Autodesk Fusion 360 part; units mm, degrees
(part 4 of 12)
  arc A1641 (188.5059, 15.9968) -> (187.8959, 15.9968) centre (188.2009, 15.9968) ccw
  arc A1642 (194.7044, 9.8652) -> (195.3144, 9.8652) centre (195.0094, 9.8652) ccw
  arc A1643 (195.3144, 9.8652) -> (194.7044, 9.8652) centre (195.0094, 9.8652) ccw
  arc A1644 (37.157, 59.1472) -> (37.767, 59.1472) centre (37.462, 59.1472) ccw
  arc A1645 (37.767, 59.1472) -> (37.157, 59.1472) centre (37.462, 59.1472) ccw
  arc A1646 (172.2547, 3.3052) -> (171.6447, 3.3052) centre (171.9497, 3.3052) ccw
  arc A1647 (171.6447, 3.3052) -> (172.2547, 3.3052) centre (171.9497, 3.3052) ccw
  arc A1648 (19.3498, 20.1403) -> (19.9598, 20.1403) centre (19.6548, 20.1403) ccw
  arc A1649 (19.9598, 20.1403) -> (19.3498, 20.1403) centre (19.6548, 20.1403) ccw
  arc A1650 (196.076, 32.2079) -> (196.686, 32.2079) centre (196.381, 32.2079) ccw
  arc A1651 (196.686, 32.2079) -> (196.076, 32.2079) centre (196.381, 32.2079) ccw
  arc A1652 (65.3089, -31.7901) -> (65.9189, -31.7901) centre (65.6139, -31.7901) ccw
  arc A1653 (65.9189, -31.7901) -> (65.3089, -31.7901) centre (65.6139, -31.7901) ccw
  arc A1654 (100.1137, 28.1421) -> (99.5037, 28.1421) centre (99.8087, 28.1421) ccw
  arc A1655 (99.5037, 28.1421) -> (100.1137, 28.1421) centre (99.8087, 28.1421) ccw
  arc A1656 (38.7626, 74.6874) -> (39.3726, 74.6874) centre (39.0676, 74.6874) ccw
  arc A1657 (39.3726, 74.6874) -> (38.7626, 74.6874) centre (39.0676, 74.6874) ccw
  arc A1658 (68.1725, 81.757) -> (68.7825, 81.757) centre (68.4775, 81.757) ccw
  arc A1659 (68.7825, 81.757) -> (68.1725, 81.757) centre (68.4775, 81.757) ccw
  arc A1660 (98.8111, 74.853) -> (99.4211, 74.853) centre (99.1161, 74.853) ccw
  arc A1661 (99.4211, 74.853) -> (98.8111, 74.853) centre (99.1161, 74.853) ccw
  arc A1662 (129.2833, 80.5774) -> (129.8933, 80.5774) centre (129.5883, 80.5774) ccw
  arc A1663 (129.8933, 80.5774) -> (129.2833, 80.5774) centre (129.5883, 80.5774) ccw
  arc A1664 (158.9828, 74.2089) -> (159.5928, 74.2089) centre (159.2878, 74.2089) ccw
  arc A1665 (159.5928, 74.2089) -> (158.9828, 74.2089) centre (159.2878, 74.2089) ccw
  arc A1666 (194.1649, 74.2089) -> (194.7749, 74.2089) centre (194.4699, 74.2089) ccw
  arc A1667 (194.7749, 74.2089) -> (194.1649, 74.2089) centre (194.4699, 74.2089) ccw
  arc A1668 (191.6955, 42.1421) -> (192.3055, 42.1421) centre (192.0005, 42.1421) ccw
  arc A1669 (192.3055, 42.1421) -> (191.6955, 42.1421) centre (192.0005, 42.1421) ccw
  arc A1670 (214.7839, 42.1421) -> (215.3939, 42.1421) centre (215.0889, 42.1421) ccw
  arc A1671 (215.3939, 42.1421) -> (214.7839, 42.1421) centre (215.0889, 42.1421) ccw
  arc A1672 (74.5184, 16.8462) -> (73.9084, 16.8462) centre (74.2134, 16.8462) ccw
  arc A1673 (73.9084, 16.8462) -> (74.5184, 16.8462) centre (74.2134, 16.8462) ccw
  arc A1674 (109.4184, 19.9249) -> (110.0284, 19.9249) centre (109.7234, 19.9249) ccw
  arc A1675 (110.0284, 19.9249) -> (109.4184, 19.9249) centre (109.7234, 19.9249) ccw
  arc A1676 (180.1512, -15.9405) -> (180.7612, -15.9405) centre (180.4562, -15.9405) ccw
  arc A1677 (180.7612, -15.9405) -> (180.1512, -15.9405) centre (180.4562, -15.9405) ccw
  arc A1678 (206.6439, -9.7413) -> (207.2539, -9.7413) centre (206.9489, -9.7413) ccw
  arc A1679 (207.2539, -9.7413) -> (206.6439, -9.7413) centre (206.9489, -9.7413) ccw
  arc A1680 (100.8626, -25.7268) -> (101.4726, -25.7268) centre (101.1676, -25.7268) ccw
  arc A1681 (101.4726, -25.7268) -> (100.8626, -25.7268) centre (101.1676, -25.7268) ccw
  line L279 (39.8781, 79.4042) -> (43.6781, 79.4042)
  line L280 (43.6781, 79.4042) -> (43.6781, 75.6042)
  line L281 (43.6781, 75.6042) -> (39.8781, 75.6042)
  line L282 (39.8781, 75.6042) -> (39.8781, 79.4042)
  arc A1682 (39.6622, 82.1982) -> (43.65, 82.1982) centre (41.6561, 82.1982) ccw
  arc A1683 (43.65, 82.1982) -> (39.6622, 82.1982) centre (41.6561, 82.1982) ccw
  arc A1684 (47.587, 82.0712) -> (45.8852, 82.0712) centre (46.7361, 82.0712) ccw
  arc A1685 (45.8852, 82.0712) -> (47.587, 82.0712) centre (46.7361, 82.0712) ccw
  arc A1686 (37.427, 82.0712) -> (35.7252, 82.0712) centre (36.5761, 82.0712) ccw
  arc A1687 (35.7252, 82.0712) -> (37.427, 82.0712) centre (36.5761, 82.0712) ccw
  line L283 (69.8781, 79.4042) -> (73.6781, 79.4042)
  line L284 (69.8781, 75.6042) -> (69.8781, 79.4042)
  line L285 (73.6781, 75.6042) -> (69.8781, 75.6042)
  line L286 (73.6781, 79.4042) -> (73.6781, 75.6042)
  arc A1688 (69.6622, 82.1982) -> (73.65, 82.1982) centre (71.6561, 82.1982) ccw
  arc A1689 (73.65, 82.1982) -> (69.6622, 82.1982) centre (71.6561, 82.1982) ccw
  arc A1690 (75.8852, 82.0712) -> (77.587, 82.0712) centre (76.7361, 82.0712) ccw
  arc A1691 (77.587, 82.0712) -> (75.8852, 82.0712) centre (76.7361, 82.0712) ccw
  arc A1692 (65.7252, 82.0712) -> (67.427, 82.0712) centre (66.5761, 82.0712) ccw
  arc A1693 (67.427, 82.0712) -> (65.7252, 82.0712) centre (66.5761, 82.0712) ccw
  line L287 (99.8781, 79.4042) -> (103.6781, 79.4042)
  line L288 (103.6781, 79.4042) -> (103.6781, 75.6042)
  line L289 (103.6781, 75.6042) -> (99.8781, 75.6042)
  line L290 (99.8781, 75.6042) -> (99.8781, 79.4042)
  arc A1694 (99.6622, 82.1982) -> (103.65, 82.1982) centre (101.6561, 82.1982) ccw
  arc A1695 (103.65, 82.1982) -> (99.6622, 82.1982) centre (101.6561, 82.1982) ccw
  arc A1696 (105.8852, 82.0712) -> (107.587, 82.0712) centre (106.7361, 82.0712) ccw
  arc A1697 (107.587, 82.0712) -> (105.8852, 82.0712) centre (106.7361, 82.0712) ccw
  arc A1698 (95.7252, 82.0712) -> (97.427, 82.0712) centre (96.5761, 82.0712) ccw
  arc A1699 (97.427, 82.0712) -> (95.7252, 82.0712) centre (96.5761, 82.0712) ccw
  line L291 (133.6781, 79.4042) -> (133.6781, 75.6042)
  line L292 (133.6781, 75.6042) -> (129.8781, 75.6042)
  line L293 (129.8781, 75.6042) -> (129.8781, 79.4042)
  line L294 (129.8781, 79.4042) -> (133.6781, 79.4042)
  arc A1700 (129.6622, 82.1982) -> (133.65, 82.1982) centre (131.6561, 82.1982) ccw
  arc A1701 (133.65, 82.1982) -> (129.6622, 82.1982) centre (131.6561, 82.1982) ccw
  arc A1702 (135.8852, 82.0712) -> (137.587, 82.0712) centre (136.7361, 82.0712) ccw
  arc A1703 (137.587, 82.0712) -> (135.8852, 82.0712) centre (136.7361, 82.0712) ccw
  arc A1704 (125.7252, 82.0712) -> (127.427, 82.0712) centre (126.5761, 82.0712) ccw
  arc A1705 (127.427, 82.0712) -> (125.7252, 82.0712) centre (126.5761, 82.0712) ccw
  line L295 (159.8781, 79.4042) -> (163.6781, 79.4042)
  line L296 (163.6781, 79.4042) -> (163.6781, 75.6042)
  line L297 (163.6781, 75.6042) -> (159.8781, 75.6042)
  line L298 (159.8781, 75.6042) -> (159.8781, 79.4042)
  arc A1706 (159.6622, 82.1982) -> (163.65, 82.1982) centre (161.6561, 82.1982) ccw
  arc A1707 (163.65, 82.1982) -> (159.6622, 82.1982) centre (161.6561, 82.1982) ccw
  arc A1708 (165.8852, 82.0712) -> (167.587, 82.0712) centre (166.7361, 82.0712) ccw
  arc A1709 (167.587, 82.0712) -> (165.8852, 82.0712) centre (166.7361, 82.0712) ccw
  arc A1710 (157.427, 82.0712) -> (155.7252, 82.0712) centre (156.5761, 82.0712) ccw
  arc A1711 (155.7252, 82.0712) -> (157.427, 82.0712) centre (156.5761, 82.0712) ccw
  line L299 (193.6781, 79.4042) -> (193.6781, 75.6042)
  line L300 (193.6781, 75.6042) -> (189.8781, 75.6042)
  line L301 (189.8781, 75.6042) -> (189.8781, 79.4042)
  line L302 (189.8781, 79.4042) -> (193.6781, 79.4042)
  arc A1712 (189.6622, 82.1982) -> (193.65, 82.1982) centre (191.6561, 82.1982) ccw
  arc A1713 (193.65, 82.1982) -> (189.6622, 82.1982) centre (191.6561, 82.1982) ccw
  arc A1714 (195.8852, 82.0712) -> (197.587, 82.0712) centre (196.7361, 82.0712) ccw
  arc A1715 (197.587, 82.0712) -> (195.8852, 82.0712) centre (196.7361, 82.0712) ccw
  arc A1716 (187.427, 82.0712) -> (185.7252, 82.0712) centre (186.5761, 82.0712) ccw
  arc A1717 (185.7252, 82.0712) -> (187.427, 82.0712) centre (186.5761, 82.0712) ccw
  line L303 (223.6781, 75.6042) -> (219.8781, 75.6042)
  line L304 (219.8781, 75.6042) -> (219.8781, 79.4042)
  line L305 (223.6781, 79.4042) -> (223.6781, 75.6042)
  line L306 (219.8781, 79.4042) -> (223.6781, 79.4042)
  arc A1718 (219.6622, 82.1982) -> (223.65, 82.1982) centre (221.6561, 82.1982) ccw
  arc A1719 (223.65, 82.1982) -> (219.6622, 82.1982) centre (221.6561, 82.1982) ccw
  arc A1720 (225.8852, 82.0712) -> (227.587, 82.0712) centre (226.7361, 82.0712) ccw
  arc A1721 (227.587, 82.0712) -> (225.8852, 82.0712) centre (226.7361, 82.0712) ccw
  arc A1722 (215.7252, 82.0712) -> (217.427, 82.0712) centre (216.5761, 82.0712) ccw
  arc A1723 (217.427, 82.0712) -> (215.7252, 82.0712) centre (216.5761, 82.0712) ccw
  line L307 (39.8781, 49.4042) -> (43.6781, 49.4042)
  line L308 (43.6781, 49.4042) -> (43.6781, 45.6042)
  line L309 (43.6781, 45.6042) -> (39.8781, 45.6042)
  line L310 (39.8781, 45.6042) -> (39.8781, 49.4042)
  arc A1724 (43.65, 52.1982) -> (39.6622, 52.1982) centre (41.6561, 52.1982) ccw
  arc A1725 (39.6622, 52.1982) -> (43.65, 52.1982) centre (41.6561, 52.1982) ccw
  arc A1726 (45.8852, 52.0712) -> (47.587, 52.0712) centre (46.7361, 52.0712) ccw
  arc A1727 (47.587, 52.0712) -> (45.8852, 52.0712) centre (46.7361, 52.0712) ccw
  arc A1728 (35.7252, 52.0712) -> (37.427, 52.0712) centre (36.5761, 52.0712) ccw
  arc A1729 (37.427, 52.0712) -> (35.7252, 52.0712) centre (36.5761, 52.0712) ccw
  line L311 (69.8781, 49.4042) -> (73.6781, 49.4042)
  line L312 (73.6781, 49.4042) -> (73.6781, 45.6042)
  line L313 (69.8781, 45.6042) -> (69.8781, 49.4042)
  line L314 (73.6781, 45.6042) -> (69.8781, 45.6042)
  arc A1730 (69.6622, 52.1982) -> (73.65, 52.1982) centre (71.6561, 52.1982) ccw
  arc A1731 (73.65, 52.1982) -> (69.6622, 52.1982) centre (71.6561, 52.1982) ccw
  arc A1732 (75.8852, 52.0712) -> (77.587, 52.0712) centre (76.7361, 52.0712) ccw
  arc A1733 (77.587, 52.0712) -> (75.8852, 52.0712) centre (76.7361, 52.0712) ccw
  arc A1734 (65.7252, 52.0712) -> (67.427, 52.0712) centre (66.5761, 52.0712) ccw
  arc A1735 (67.427, 52.0712) -> (65.7252, 52.0712) centre (66.5761, 52.0712) ccw
  line L315 (99.8781, 45.6042) -> (99.8781, 49.4042)
  line L316 (99.8781, 49.4042) -> (103.6781, 49.4042)
  line L317 (103.6781, 49.4042) -> (103.6781, 45.6042)
  line L318 (103.6781, 45.6042) -> (99.8781, 45.6042)
  arc A1736 (99.6622, 52.1982) -> (103.65, 52.1982) centre (101.6561, 52.1982) ccw
  arc A1737 (103.65, 52.1982) -> (99.6622, 52.1982) centre (101.6561, 52.1982) ccw
  arc A1738 (105.8852, 52.0712) -> (107.587, 52.0712) centre (106.7361, 52.0712) ccw
  arc A1739 (107.587, 52.0712) -> (105.8852, 52.0712) centre (106.7361, 52.0712) ccw
  arc A1740 (95.7252, 52.0712) -> (97.427, 52.0712) centre (96.5761, 52.0712) ccw
  arc A1741 (97.427, 52.0712) -> (95.7252, 52.0712) centre (96.5761, 52.0712) ccw
  line L319 (129.8781, 49.4042) -> (133.6781, 49.4042)
  line L320 (133.6781, 49.4042) -> (133.6781, 45.6042)
  line L321 (133.6781, 45.6042) -> (129.8781, 45.6042)
  line L322 (129.8781, 45.6042) -> (129.8781, 49.4042)
  arc A1742 (129.6622, 52.1982) -> (133.65, 52.1982) centre (131.6561, 52.1982) ccw
  arc A1743 (133.65, 52.1982) -> (129.6622, 52.1982) centre (131.6561, 52.1982) ccw
  arc A1744 (135.8852, 52.0712) -> (137.587, 52.0712) centre (136.7361, 52.0712) ccw
  arc A1745 (137.587, 52.0712) -> (135.8852, 52.0712) centre (136.7361, 52.0712) ccw
  arc A1746 (125.7252, 52.0712) -> (127.427, 52.0712) centre (126.5761, 52.0712) ccw
  arc A1747 (127.427, 52.0712) -> (125.7252, 52.0712) centre (126.5761, 52.0712) ccw
  line L323 (159.8781, 45.6042) -> (159.8781, 49.4042)
  line L324 (163.6781, 45.6042) -> (159.8781, 45.6042)
  line L325 (163.6781, 49.4042) -> (163.6781, 45.6042)
  line L326 (159.8781, 49.4042) -> (163.6781, 49.4042)
  arc A1748 (159.6622, 52.1982) -> (163.65, 52.1982) centre (161.6561, 52.1982) ccw
  arc A1749 (163.65, 52.1982) -> (159.6622, 52.1982) centre (161.6561, 52.1982) ccw
  arc A1750 (165.8852, 52.0712) -> (167.587, 52.0712) centre (166.7361, 52.0712) ccw
  arc A1751 (167.587, 52.0712) -> (165.8852, 52.0712) centre (166.7361, 52.0712) ccw
  arc A1752 (155.7252, 52.0712) -> (157.427, 52.0712) centre (156.5761, 52.0712) ccw
  arc A1753 (157.427, 52.0712) -> (155.7252, 52.0712) centre (156.5761, 52.0712) ccw
  line L327 (189.8781, 49.4042) -> (193.6781, 49.4042)
  line L328 (193.6781, 49.4042) -> (193.6781, 45.6042)
  line L329 (193.6781, 45.6042) -> (189.8781, 45.6042)
  line L330 (189.8781, 45.6042) -> (189.8781, 49.4042)
  arc A1754 (189.6622, 52.1982) -> (193.65, 52.1982) centre (191.6561, 52.1982) ccw
  arc A1755 (193.65, 52.1982) -> (189.6622, 52.1982) centre (191.6561, 52.1982) ccw
  arc A1756 (195.8852, 52.0712) -> (197.587, 52.0712) centre (196.7361, 52.0712) ccw
  arc A1757 (197.587, 52.0712) -> (195.8852, 52.0712) centre (196.7361, 52.0712) ccw
  arc A1758 (185.7252, 52.0712) -> (187.427, 52.0712) centre (186.5761, 52.0712) ccw
  arc A1759 (187.427, 52.0712) -> (185.7252, 52.0712) centre (186.5761, 52.0712) ccw
  line L331 (219.8781, 49.4042) -> (223.6781, 49.4042)
  line L332 (223.6781, 49.4042) -> (223.6781, 45.6042)
  line L333 (223.6781, 45.6042) -> (219.8781, 45.6042)
  line L334 (219.8781, 45.6042) -> (219.8781, 49.4042)
  arc A1760 (223.65, 52.1982) -> (219.6622, 52.1982) centre (221.6561, 52.1982) ccw
  arc A1761 (219.6622, 52.1982) -> (223.65, 52.1982) centre (221.6561, 52.1982) ccw
  arc A1762 (225.8852, 52.0712) -> (227.587, 52.0712) centre (226.7361, 52.0712) ccw
  arc A1763 (227.587, 52.0712) -> (225.8852, 52.0712) centre (226.7361, 52.0712) ccw
  arc A1764 (215.7252, 52.0712) -> (217.427, 52.0712) centre (216.5761, 52.0712) ccw
  arc A1765 (217.427, 52.0712) -> (215.7252, 52.0712) centre (216.5761, 52.0712) ccw
  line L335 (39.8781, 19.4042) -> (43.6781, 19.4042)
  line L336 (39.8781, 15.6042) -> (39.8781, 19.4042)
  line L337 (43.6781, 19.4042) -> (43.6781, 15.6042)
  line L338 (43.6781, 15.6042) -> (39.8781, 15.6042)
  arc A1766 (43.65, 22.1982) -> (39.6622, 22.1982) centre (41.6561, 22.1982) ccw
  arc A1767 (39.6622, 22.1982) -> (43.65, 22.1982) centre (41.6561, 22.1982) ccw
  arc A1768 (45.8852, 22.0712) -> (47.587, 22.0712) centre (46.7361, 22.0712) ccw
  arc A1769 (47.587, 22.0712) -> (45.8852, 22.0712) centre (46.7361, 22.0712) ccw
  arc A1770 (35.7252, 22.0712) -> (37.427, 22.0712) centre (36.5761, 22.0712) ccw
  arc A1771 (37.427, 22.0712) -> (35.7252, 22.0712) centre (36.5761, 22.0712) ccw
  line L339 (75.9614, 19.4601) -> (79.7614, 19.4601)
  line L340 (79.7614, 19.4601) -> (79.7614, 15.6601)
  line L341 (79.7614, 15.6601) -> (75.9614, 15.6601)
  line L342 (75.9614, 15.6601) -> (75.9614, 19.4601)
  arc A1772 (79.7333, 22.2541) -> (75.7455, 22.2541) centre (77.7394, 22.2541) ccw
  arc A1773 (75.7455, 22.2541) -> (79.7333, 22.2541) centre (77.7394, 22.2541) ccw
  arc A1774 (83.6703, 22.1271) -> (81.9685, 22.1271) centre (82.8194, 22.1271) ccw
  arc A1775 (81.9685, 22.1271) -> (83.6703, 22.1271) centre (82.8194, 22.1271) ccw
  arc A1776 (71.8085, 22.1271) -> (73.5103, 22.1271) centre (72.6594, 22.1271) ccw
  arc A1777 (73.5103, 22.1271) -> (71.8085, 22.1271) centre (72.6594, 22.1271) ccw
  line L343 (105.9614, 19.4601) -> (109.7614, 19.4601)
  line L344 (109.7614, 19.4601) -> (109.7614, 15.6601)
  line L345 (109.7614, 15.6601) -> (105.9614, 15.6601)
  line L346 (105.9614, 15.6601) -> (105.9614, 19.4601)
  arc A1778 (105.7455, 22.2541) -> (109.7333, 22.2541) centre (107.7394, 22.2541) ccw
  arc A1779 (109.7333, 22.2541) -> (105.7455, 22.2541) centre (107.7394, 22.2541) ccw
  arc A1780 (113.6703, 22.1271) -> (111.9685, 22.1271) centre (112.8194, 22.1271) ccw
  arc A1781 (111.9685, 22.1271) -> (113.6703, 22.1271) centre (112.8194, 22.1271) ccw
  arc A1782 (103.5103, 22.1271) -> (101.8085, 22.1271) centre (102.6594, 22.1271) ccw
  arc A1783 (101.8085, 22.1271) -> (103.5103, 22.1271) centre (102.6594, 22.1271) ccw
  line L347 (135.9614, 19.4601) -> (139.7614, 19.4601)
  line L348 (135.9614, 15.6601) -> (135.9614, 19.4601)
  line L349 (139.7614, 15.6601) -> (135.9614, 15.6601)
  line L350 (139.7614, 19.4601) -> (139.7614, 15.6601)
  arc A1784 (135.7455, 22.2541) -> (139.7333, 22.2541) centre (137.7394, 22.2541) ccw
  arc A1785 (139.7333, 22.2541) -> (135.7455, 22.2541) centre (137.7394, 22.2541) ccw
  arc A1786 (141.9685, 22.1271) -> (143.6703, 22.1271) centre (142.8194, 22.1271) ccw
  arc A1787 (143.6703, 22.1271) -> (141.9685, 22.1271) centre (142.8194, 22.1271) ccw
  arc A1788 (131.8085, 22.1271) -> (133.5103, 22.1271) centre (132.6594, 22.1271) ccw
  arc A1789 (133.5103, 22.1271) -> (131.8085, 22.1271) centre (132.6594, 22.1271) ccw
  line L351 (165.9614, 19.4601) -> (169.7614, 19.4601)
  line L352 (169.7614, 19.4601) -> (169.7614, 15.6601)
  line L353 (169.7614, 15.6601) -> (165.9614, 15.6601)
  line L354 (165.9614, 15.6601) -> (165.9614, 19.4601)
  arc A1790 (165.7455, 22.2541) -> (169.7333, 22.2541) centre (167.7394, 22.2541) ccw
  arc A1791 (169.7333, 22.2541) -> (165.7455, 22.2541) centre (167.7394, 22.2541) ccw
  arc A1792 (171.9685, 22.1271) -> (173.6703, 22.1271) centre (172.8194, 22.1271) ccw
  arc A1793 (173.6703, 22.1271) -> (171.9685, 22.1271) centre (172.8194, 22.1271) ccw
  arc A1794 (161.8085, 22.1271) -> (163.5103, 22.1271) centre (162.6594, 22.1271) ccw
  arc A1795 (163.5103, 22.1271) -> (161.8085, 22.1271) centre (162.6594, 22.1271) ccw
  line L355 (195.9614, 19.4601) -> (199.7614, 19.4601)
  line L356 (199.7614, 19.4601) -> (199.7614, 15.6601)
  line L357 (199.7614, 15.6601) -> (195.9614, 15.6601)
  line L358 (195.9614, 15.6601) -> (195.9614, 19.4601)
  arc A1796 (199.7333, 22.2541) -> (195.7455, 22.2541) centre (197.7394, 22.2541) ccw
  arc A1797 (195.7455, 22.2541) -> (199.7333, 22.2541) centre (197.7394, 22.2541) ccw
  arc A1798 (203.6703, 22.1271) -> (201.9685, 22.1271) centre (202.8194, 22.1271) ccw
  arc A1799 (201.9685, 22.1271) -> (203.6703, 22.1271) centre (202.8194, 22.1271) ccw
  arc A1800 (191.8085, 22.1271) -> (193.5103, 22.1271) centre (192.6594, 22.1271) ccw
  arc A1801 (193.5103, 22.1271) -> (191.8085, 22.1271) centre (192.6594, 22.1271) ccw
  line L359 (114.6812, -67.9859) -> (118.4812, -67.9859)
  line L360 (118.4812, -67.9859) -> (118.4812, -71.7859)
  line L361 (118.4812, -71.7859) -> (114.6812, -71.7859)
  line L362 (114.6812, -71.7859) -> (114.6812, -67.9859)
  arc A1802 (114.4653, -65.1919) -> (118.4531, -65.1919) centre (116.4592, -65.1919) ccw
  arc A1803 (118.4531, -65.1919) -> (114.4653, -65.1919) centre (116.4592, -65.1919) ccw
  arc A1804 (120.6883, -65.3189) -> (122.3901, -65.3189) centre (121.5392, -65.3189) ccw
  arc A1805 (122.3901, -65.3189) -> (120.6883, -65.3189) centre (121.5392, -65.3189) ccw
  arc A1806 (110.5283, -65.3189) -> (112.2301, -65.3189) centre (111.3792, -65.3189) ccw
  arc A1807 (112.2301, -65.3189) -> (110.5283, -65.3189) centre (111.3792, -65.3189) ccw
  line L363 (39.8781, -10.5958) -> (43.6781, -10.5958)
  line L364 (43.6781, -10.5958) -> (43.6781, -14.3958)
  line L365 (43.6781, -14.3958) -> (39.8781, -14.3958)
  line L366 (39.8781, -14.3958) -> (39.8781, -10.5958)
  arc A1808 (39.6622, -7.8018) -> (43.65, -7.8018) centre (41.6561, -7.8018) ccw
  arc A1809 (43.65, -7.8018) -> (39.6622, -7.8018) centre (41.6561, -7.8018) ccw
  arc A1810 (47.587, -7.9288) -> (45.8852, -7.9288) centre (46.7361, -7.9288) ccw
  arc A1811 (45.8852, -7.9288) -> (47.587, -7.9288) centre (46.7361, -7.9288) ccw
  arc A1812 (35.7252, -7.9288) -> (37.427, -7.9288) centre (36.5761, -7.9288) ccw
  arc A1813 (37.427, -7.9288) -> (35.7252, -7.9288) centre (36.5761, -7.9288) ccw
  line L367 (86.8834, -10.639) -> (90.6834, -10.639)
  line L368 (90.6834, -14.439) -> (86.8834, -14.439)
  line L369 (86.8834, -14.439) -> (86.8834, -10.639)
  line L370 (90.6834, -10.639) -> (90.6834, -14.439)
  arc A1814 (90.6553, -7.845) -> (86.6675, -7.845) centre (88.6614, -7.845) ccw
  arc A1815 (86.6675, -7.845) -> (90.6553, -7.845) centre (88.6614, -7.845) ccw
  arc A1816 (92.8905, -7.972) -> (94.5923, -7.972) centre (93.7414, -7.972) ccw
  arc A1817 (94.5923, -7.972) -> (92.8905, -7.972) centre (93.7414, -7.972) ccw
  arc A1818 (82.7305, -7.972) -> (84.4323, -7.972) centre (83.5814, -7.972) ccw
  arc A1819 (84.4323, -7.972) -> (82.7305, -7.972) centre (83.5814, -7.972) ccw
  line L371 (116.8834, -10.639) -> (120.6834, -10.639)
  line L372 (120.6834, -10.639) -> (120.6834, -14.439)
  line L373 (120.6834, -14.439) -> (116.8834, -14.439)
  line L374 (116.8834, -14.439) -> (116.8834, -10.639)
  arc A1820 (116.6675, -7.845) -> (120.6553, -7.845) centre (118.6614, -7.845) ccw
  arc A1821 (120.6553, -7.845) -> (116.6675, -7.845) centre (118.6614, -7.845) ccw
  arc A1822 (124.5923, -7.972) -> (122.8905, -7.972) centre (123.7414, -7.972) ccw
  arc A1823 (122.8905, -7.972) -> (124.5923, -7.972) centre (123.7414, -7.972) ccw
  arc A1824 (112.7305, -7.972) -> (114.4323, -7.972) centre (113.5814, -7.972) ccw
  arc A1825 (114.4323, -7.972) -> (112.7305, -7.972) centre (113.5814, -7.972) ccw
  line L375 (146.8834, -10.639) -> (150.6834, -10.639)
  line L376 (150.6834, -10.639) -> (150.6834, -14.439)
  line L377 (150.6834, -14.439) -> (146.8834, -14.439)
  line L378 (146.8834, -14.439) -> (146.8834, -10.639)
  arc A1826 (146.6675, -7.845) -> (150.6553, -7.845) centre (148.6614, -7.845) ccw
  arc A1827 (150.6553, -7.845) -> (146.6675, -7.845) centre (148.6614, -7.845) ccw
  arc A1828 (154.5923, -7.972) -> (152.8905, -7.972) centre (153.7414, -7.972) ccw
  arc A1829 (152.8905, -7.972) -> (154.5923, -7.972) centre (153.7414, -7.972) ccw
  arc A1830 (144.4323, -7.972) -> (142.7305, -7.972) centre (143.5814, -7.972) ccw
  arc A1831 (142.7305, -7.972) -> (144.4323, -7.972) centre (143.5814, -7.972) ccw
  line L379 (176.8834, -10.639) -> (180.6834, -10.639)
  line L380 (180.6834, -10.639) -> (180.6834, -14.439)
  line L381 (180.6834, -14.439) -> (176.8834, -14.439)
  line L382 (176.8834, -14.439) -> (176.8834, -10.639)
  arc A1832 (176.6675, -7.845) -> (180.6553, -7.845) centre (178.6614, -7.845) ccw
  arc A1833 (180.6553, -7.845) -> (176.6675, -7.845) centre (178.6614, -7.845) ccw
  arc A1834 (182.8905, -7.972) -> (184.5923, -7.972) centre (183.7414, -7.972) ccw
  arc A1835 (184.5923, -7.972) -> (182.8905, -7.972) centre (183.7414, -7.972) ccw
  arc A1836 (172.7305, -7.972) -> (174.4323, -7.972) centre (173.5814, -7.972) ccw
  arc A1837 (174.4323, -7.972) -> (172.7305, -7.972) centre (173.5814, -7.972) ccw
  line L383 (210.6834, -10.639) -> (210.6834, -14.439)
  line L384 (206.8834, -14.439) -> (206.8834, -10.639)
  line L385 (206.8834, -10.639) -> (210.6834, -10.639)
  line L386 (210.6834, -14.439) -> (206.8834, -14.439)
  arc A1838 (206.6675, -7.845) -> (210.6553, -7.845) centre (208.6614, -7.845) ccw
  arc A1839 (210.6553, -7.845) -> (206.6675, -7.845) centre (208.6614, -7.845) ccw
  arc A1840 (212.8905, -7.972) -> (214.5923, -7.972) centre (213.7414, -7.972) ccw
  arc A1841 (214.5923, -7.972) -> (212.8905, -7.972) centre (213.7414, -7.972) ccw
  arc A1842 (202.7305, -7.972) -> (204.4323, -7.972) centre (203.5814, -7.972) ccw
  arc A1843 (204.4323, -7.972) -> (202.7305, -7.972) centre (203.5814, -7.972) ccw
  line L387 (158.7503, -71.7859) -> (158.7503, -67.9859)
  line L388 (162.5503, -71.7859) -> (158.7503, -71.7859)
  line L389 (162.5503, -67.9859) -> (162.5503, -71.7859)
  line L390 (158.7503, -67.9859) -> (162.5503, -67.9859)
  arc A1844 (158.5344, -65.1919) -> (162.5222, -65.1919) centre (160.5283, -65.1919) ccw
  arc A1845 (162.5222, -65.1919) -> (158.5344, -65.1919) centre (160.5283, -65.1919) ccw
  arc A1846 (164.7574, -65.3189) -> (166.4592, -65.3189) centre (165.6083, -65.3189) ccw
  arc A1847 (166.4592, -65.3189) -> (164.7574, -65.3189) centre (165.6083, -65.3189) ccw
  arc A1848 (154.5974, -65.3189) -> (156.2992, -65.3189) centre (155.4483, -65.3189) ccw
  arc A1849 (156.2992, -65.3189) -> (154.5974, -65.3189) centre (155.4483, -65.3189) ccw
  line L391 (39.8781, -40.5958) -> (43.6781, -40.5958)
  line L392 (43.6781, -40.5958) -> (43.6781, -44.3958)
  line L393 (43.6781, -44.3958) -> (39.8781, -44.3958)
  line L394 (39.8781, -44.3958) -> (39.8781, -40.5958)
  arc A1850 (39.6622, -37.8018) -> (43.65, -37.8018) centre (41.6561, -37.8018) ccw
  arc A1851 (43.65, -37.8018) -> (39.6622, -37.8018) centre (41.6561, -37.8018) ccw
  arc A1852 (45.8852, -37.9288) -> (47.587, -37.9288) centre (46.7361, -37.9288) ccw
  arc A1853 (47.587, -37.9288) -> (45.8852, -37.9288) centre (46.7361, -37.9288) ccw
  arc A1854 (35.7252, -37.9288) -> (37.427, -37.9288) centre (36.5761, -37.9288) ccw
  arc A1855 (37.427, -37.9288) -> (35.7252, -37.9288) centre (36.5761, -37.9288) ccw
  line L395 (96.4084, -40.611) -> (100.2084, -40.611)
  line L396 (100.2084, -40.611) -> (100.2084, -44.411)
  line L397 (100.2084, -44.411) -> (96.4084, -44.411)
  line L398 (96.4084, -44.411) -> (96.4084, -40.611)
  arc A1856 (96.1925, -37.817) -> (100.1803, -37.817) centre (98.1864, -37.817) ccw
  arc A1857 (100.1803, -37.817) -> (96.1925, -37.817) centre (98.1864, -37.817) ccw
  arc A1858 (102.4155, -37.944) -> (104.1173, -37.944) centre (103.2664, -37.944) ccw
  arc A1859 (104.1173, -37.944) -> (102.4155, -37.944) centre (103.2664, -37.944) ccw
  arc A1860 (92.2555, -37.944) -> (93.9573, -37.944) centre (93.1064, -37.944) ccw
  arc A1861 (93.9573, -37.944) -> (92.2555, -37.944) centre (93.1064, -37.944) ccw
  line L399 (126.4084, -40.611) -> (130.2084, -40.611)
  line L400 (130.2084, -40.611) -> (130.2084, -44.411)
  line L401 (130.2084, -44.411) -> (126.4084, -44.411)
  line L402 (126.4084, -44.411) -> (126.4084, -40.611)
  arc A1862 (126.1925, -37.817) -> (130.1803, -37.817) centre (128.1864, -37.817) ccw
  arc A1863 (130.1803, -37.817) -> (126.1925, -37.817) centre (128.1864, -37.817) ccw
  arc A1864 (132.4155, -37.944) -> (134.1173, -37.944) centre (133.2664, -37.944) ccw
  arc A1865 (134.1173, -37.944) -> (132.4155, -37.944) centre (133.2664, -37.944) ccw
  arc A1866 (122.2555, -37.944) -> (123.9573, -37.944) centre (123.1064, -37.944) ccw
  arc A1867 (123.9573, -37.944) -> (122.2555, -37.944) centre (123.1064, -37.944) ccw
  line L403 (160.2084, -44.411) -> (156.4084, -44.411)
  line L404 (160.2084, -40.611) -> (160.2084, -44.411)
  line L405 (156.4084, -40.611) -> (160.2084, -40.611)
  line L406 (156.4084, -44.411) -> (156.4084, -40.611)
  arc A1868 (156.1925, -37.817) -> (160.1803, -37.817) centre (158.1864, -37.817) ccw
  arc A1869 (160.1803, -37.817) -> (156.1925, -37.817) centre (158.1864, -37.817) ccw
  arc A1870 (162.4155, -37.944) -> (164.1173, -37.944) centre (163.2664, -37.944) ccw
  arc A1871 (164.1173, -37.944) -> (162.4155, -37.944) centre (163.2664, -37.944) ccw
  arc A1872 (152.2555, -37.944) -> (153.9573, -37.944) centre (153.1064, -37.944) ccw
  arc A1873 (153.9573, -37.944) -> (152.2555, -37.944) centre (153.1064, -37.944) ccw
  line L407 (186.4084, -40.611) -> (190.2084, -40.611)
  line L408 (190.2084, -40.611) -> (190.2084, -44.411)
  line L409 (190.2084, -44.411) -> (186.4084, -44.411)
  line L410 (186.4084, -44.411) -> (186.4084, -40.611)
  arc A1874 (186.1925, -37.817) -> (190.1803, -37.817) centre (188.1864, -37.817) ccw
  arc A1875 (190.1803, -37.817) -> (186.1925, -37.817) centre (188.1864, -37.817) ccw
  arc A1876 (192.4155, -37.944) -> (194.1173, -37.944) centre (193.2664, -37.944) ccw
  arc A1877 (194.1173, -37.944) -> (192.4155, -37.944) centre (193.2664, -37.944) ccw
  arc A1878 (182.2555, -37.944) -> (183.9573, -37.944) centre (183.1064, -37.944) ccw
  arc A1879 (183.9573, -37.944) -> (182.2555, -37.944) centre (183.1064, -37.944) ccw
  line L411 (216.4084, -40.611) -> (220.2084, -40.611)
  line L412 (216.4084, -44.411) -> (216.4084, -40.611)
  line L413 (220.2084, -44.411) -> (216.4084, -44.411)
  line L414 (220.2084, -40.611) -> (220.2084, -44.411)
  arc A1880 (216.1925, -37.817) -> (220.1803, -37.817) centre (218.1864, -37.817) ccw
  arc A1881 (220.1803, -37.817) -> (216.1925, -37.817) centre (218.1864, -37.817) ccw
  arc A1882 (222.4155, -37.944) -> (224.1173, -37.944) centre (223.2664, -37.944) ccw
  arc A1883 (224.1173, -37.944) -> (222.4155, -37.944) centre (223.2664, -37.944) ccw
  arc A1884 (212.2555, -37.944) -> (213.9573, -37.944) centre (213.1064, -37.944) ccw
  arc A1885 (213.9573, -37.944) -> (212.2555, -37.944) centre (213.1064, -37.944) ccw
  line L415 (203.2004, -67.9859) -> (207.0004, -67.9859)
  line L416 (207.0004, -67.9859) -> (207.0004, -71.7859)
  line L417 (207.0004, -71.7859) -> (203.2004, -71.7859)
  line L418 (203.2004, -71.7859) -> (203.2004, -67.9859)
  arc A1886 (202.9845, -65.1919) -> (206.9723, -65.1919) centre (204.9784, -65.1919) ccw
  arc A1887 (206.9723, -65.1919) -> (202.9845, -65.1919) centre (204.9784, -65.1919) ccw
  arc A1888 (209.2075, -65.3189) -> (210.9093, -65.3189) centre (210.0584, -65.3189) ccw
  arc A1889 (210.9093, -65.3189) -> (209.2075, -65.3189) centre (210.0584, -65.3189) ccw
  arc A1890 (199.0475, -65.3189) -> (200.7493, -65.3189) centre (199.8984, -65.3189) ccw
  arc A1891 (200.7493, -65.3189) -> (199.0475, -65.3189) centre (199.8984, -65.3189) ccw
  line L419 (43.6781, -71.7859) -> (39.8781, -71.7859)
  line L420 (43.6781, -67.9859) -> (43.6781, -71.7859)
  line L421 (39.8781, -67.9859) -> (43.6781, -67.9859)
  line L422 (39.8781, -71.7859) -> (39.8781, -67.9859)
  arc A1892 (39.6622, -65.1919) -> (43.65, -65.1919) centre (41.6561, -65.1919) ccw
  arc A1893 (43.65, -65.1919) -> (39.6622, -65.1919) centre (41.6561, -65.1919) ccw
  arc A1894 (45.8852, -65.3189) -> (47.587, -65.3189) centre (46.7361, -65.3189) ccw
  arc A1895 (47.587, -65.3189) -> (45.8852, -65.3189) centre (46.7361, -65.3189) ccw
  arc A1896 (35.7252, -65.3189) -> (37.427, -65.3189) centre (36.5761, -65.3189) ccw
  arc A1897 (37.427, -65.3189) -> (35.7252, -65.3189) centre (36.5761, -65.3189) ccw
  line L423 (74.0411, -67.9859) -> (77.8411, -67.9859)
  line L424 (77.8411, -67.9859) -> (77.8411, -71.7859)
  line L425 (77.8411, -71.7859) -> (74.0411, -71.7859)
  line L426 (74.0411, -71.7859) -> (74.0411, -67.9859)
  arc A1898 (73.8252, -65.1919) -> (77.8131, -65.1919) centre (75.8192, -65.1919) ccw
  arc A1899 (77.8131, -65.1919) -> (73.8252, -65.1919) centre (75.8192, -65.1919) ccw
  arc A1900 (80.0483, -65.3189) -> (81.7501, -65.3189) centre (80.8992, -65.3189) ccw
  arc A1901 (81.7501, -65.3189) -> (80.0483, -65.3189) centre (80.8992, -65.3189) ccw
  arc A1902 (71.59, -65.3189) -> (69.8882, -65.3189) centre (70.7391, -65.3189) ccw
  arc A1903 (69.8882, -65.3189) -> (71.59, -65.3189) centre (70.7391, -65.3189) ccw
  arc A1904 (207.6588, 87.4842) -> (206.1588, 87.4842) centre (206.9088, 87.4842) ccw
  arc A1905 (206.1588, 87.4842) -> (207.6588, 87.4842) centre (206.9088, 87.4842) ccw
  arc A1906 (207.7096, 80.4662) -> (206.2096, 80.4662) centre (206.9596, 80.4662) ccw
  arc A1907 (206.2096, 80.4662) -> (207.7096, 80.4662) centre (206.9596, 80.4662) ccw
  line L427 (-6.9407, 9.4411) -> (-6.8392, 9.492)
  line L428 (-6.8392, 9.492) -> (-6.7885, 9.6419)
  line L429 (-6.7885, 9.6419) -> (-6.7885, 9.7435)
  line L430 (-6.7885, 9.7435) -> (-6.8395, 9.8933)
  line L431 (-6.8395, 9.8933) -> (-6.9919, 9.9948)
  line L432 (-6.9919, 9.9948) -> (-7.2434, 10.0454)
  line L433 (-7.2434, 10.0454) -> (-7.4949, 10.0453)
  line L434 (-7.4949, 10.0453) -> (-7.698, 9.9943)
  line L435 (-7.698, 9.9943) -> (-7.797, 9.8926)
  line L436 (-7.797, 9.8926) -> (-7.8477, 9.7427)
  line L437 (-7.8477, 9.7427) -> (-7.8477, 9.6919)
  line L438 (-7.8477, 9.6919) -> (-7.7968, 9.5421)
  line L439 (-7.7968, 9.5421) -> (-7.6976, 9.4406)
  line L440 (-7.6976, 9.4406) -> (-7.5452, 9.3899)
  line L441 (-7.5452, 9.3899) -> (-7.4944, 9.3899)
  line L442 (-7.4944, 9.3899) -> (-7.3446, 9.4408)
  line L443 (-7.3446, 9.4408) -> (-7.2431, 9.5425)
  line L444 (-7.2431, 9.5425) -> (-7.1924, 9.6924)
  line L445 (-7.1924, 9.6924) -> (-7.1924, 9.7432)
  line L446 (-7.1924, 9.7432) -> (-7.2433, 9.893)
  line L447 (-7.2433, 9.893) -> (-7.345, 9.9946)
  line L448 (-7.345, 9.9946) -> (-7.4949, 10.0453)
  line L449 (-7.796, 8.4423) -> (-7.8469, 8.5921)
  line L450 (-6.7877, 8.5929) -> (-6.7878, 8.7961)
  line L451 (-6.9404, 8.9966) -> (-7.042, 8.9966)
  line L452 (-7.042, 8.9966) -> (-7.141, 8.9457)
  line L453 (-7.141, 8.9457) -> (-7.1917, 8.8441)
  line L454 (-7.1917, 8.8441) -> (-7.2424, 8.6434)
  line L455 (-7.2424, 8.6434) -> (-7.2931, 8.4909)
  line L456 (-7.2931, 8.4909) -> (-7.3946, 8.3918)
  line L457 (-7.3946, 8.3918) -> (-7.4936, 8.3409)
  line L458 (-7.4936, 8.3409) -> (-7.646, 8.3408)
  line L459 (-7.646, 8.3408) -> (-7.7451, 8.3915)
  line L460 (-7.7451, 8.3915) -> (-7.796, 8.4423)
  line L461 (-6.7878, 8.7961) -> (-6.8388, 8.9459)
  line L462 (-7.8469, 8.5921) -> (-7.847, 8.7953)
  line L463 (-7.847, 8.7953) -> (-7.7963, 8.9452)
  line L464 (-7.7963, 8.9452) -> (-7.7456, 8.9961)
  line L465 (-7.7456, 8.9961) -> (-7.6466, 9.0469)
  line L466 (-7.6466, 9.0469) -> (-7.4942, 9.047)
  line L467 (-7.4942, 9.047) -> (-7.3951, 8.9963)
  line L468 (-7.3951, 8.9963) -> (-7.2934, 8.8948)
  line L469 (-7.2934, 8.8948) -> (-7.2425, 8.745)
  line L470 (-7.2425, 8.745) -> (-7.1915, 8.5418)
  line L471 (-7.1915, 8.5418) -> (-7.1406, 8.4428)
  line L472 (-7.1406, 8.4428) -> (-7.0416, 8.392)
  line L473 (-7.0416, 8.392) -> (-6.94, 8.3921)
  line L474 (-6.94, 8.3921) -> (-6.8384, 8.443)
  line L475 (-6.8384, 8.443) -> (-6.7877, 8.5929)
  line L476 (-6.8388, 8.9459) -> (-6.9404, 8.9966)
  line L477 (-6.9905, 7.9984) -> (-6.9396, 7.8968)
  line L478 (-6.9396, 7.8968) -> (-6.7871, 7.7471)
  line L479 (-6.7871, 7.7471) -> (-7.8463, 7.7463)
  line L480 (-6.7866, 7.1019) -> (-6.8375, 7.2517)
  line L481 (-6.8375, 7.2517) -> (-6.99, 7.3532)
  line L482 (-6.99, 7.3532) -> (-7.2415, 7.4038)
  line L483 (-7.2415, 7.4038) -> (-7.3939, 7.4037)
  line L484 (-7.3939, 7.4037) -> (-7.6453, 7.3527)
  line L485 (-7.6453, 7.3527) -> (-7.7951, 7.251)
  line L486 (-7.7951, 7.251) -> (-7.8458, 7.1011)
  line L487 (-7.8458, 7.1011) -> (-7.8457, 6.9995)
  line L488 (-7.8457, 6.9995) -> (-7.7948, 6.8472)
  line L489 (-7.7948, 6.8472) -> (-7.6449, 6.7482)
  line L490 (-7.6449, 6.7482) -> (-7.3934, 6.6976)
  line L491 (-7.3934, 6.6976) -> (-7.241, 6.6977)
  line L492 (-7.241, 6.6977) -> (-6.9895, 6.7487)
  line L493 (-6.9895, 6.7487) -> (-6.8372, 6.8479)
  line L494 (-6.8372, 6.8479) -> (-6.7865, 7.0003)
  line L495 (-6.7865, 7.0003) -> (-6.7866, 7.1019)
  line L496 (-7.6445, 6.2529) -> (-7.5937, 6.3038)
  line L497 (-7.6446, 6.3545) -> (-7.6953, 6.3037)
  line L498 (-7.6953, 6.3037) -> (-7.6445, 6.2529)
  line L499 (-7.5937, 6.3038) -> (-7.6446, 6.3545)
  line L500 (-6.8361, 5.3544) -> (-6.7854, 5.5068)
  line L501 (-6.8364, 5.7582) -> (-6.9889, 5.8597)
  line L502 (-6.9889, 5.8597) -> (-7.2404, 5.9103)
  line L503 (-7.2404, 5.9103) -> (-7.3928, 5.9102)
  line L504 (-7.3928, 5.9102) -> (-7.6442, 5.8592)
  line L505 (-7.6442, 5.8592) -> (-7.794, 5.7575)
  line L506 (-7.794, 5.7575) -> (-7.8447, 5.6076)
  line L507 (-7.8447, 5.6076) -> (-7.8446, 5.506)
  line L508 (-7.8446, 5.506) -> (-7.7937, 5.3536)
  line L509 (-7.7937, 5.3536) -> (-7.6438, 5.2547)
  line L510 (-7.6438, 5.2547) -> (-7.3923, 5.2041)
  line L511 (-7.3923, 5.2041) -> (-7.2399, 5.2042)
  line L512 (-7.2399, 5.2042) -> (-6.9884, 5.2552)
  line L513 (-6.9884, 5.2552) -> (-6.8361, 5.3544)
  line L514 (-6.7855, 5.6084) -> (-6.8364, 5.7582)
  line L515 (-6.7854, 5.5068) -> (-6.7855, 5.6084)
  line L516 (-6.7847, 4.5594) -> (-6.8356, 4.7092)
  line L517 (-6.8356, 4.7092) -> (-6.9881, 4.8107)
  line L518 (-6.9881, 4.8107) -> (-7.2396, 4.8613)
  line L519 (-7.2396, 4.8613) -> (-7.392, 4.8612)
  line L520 (-7.392, 4.8612) -> (-7.6434, 4.8102)
  line L521 (-7.6434, 4.8102) -> (-7.7932, 4.7085)
  line L522 (-7.7932, 4.7085) -> (-7.8439, 4.5586)
  line L523 (-7.8439, 4.5586) -> (-7.8438, 4.457)
  line L524 (-7.8438, 4.457) -> (-7.7929, 4.3046)
  line L525 (-7.7929, 4.3046) -> (-7.643, 4.2057)
  line L526 (-7.643, 4.2057) -> (-7.3915, 4.1551)
  line L527 (-7.3915, 4.1551) -> (-7.2391, 4.1552)
  line L528 (-7.2391, 4.1552) -> (-6.9877, 4.2062)
  line L529 (-6.9877, 4.2062) -> (-6.8354, 4.3053)
  line L530 (-6.8354, 4.3053) -> (-6.7847, 4.4578)
  line L531 (-6.7847, 4.4578) -> (-6.7847, 4.5594)
  line L532 (-6.8857, 3.7109) -> (-6.8349, 3.6602)
  line L533 (-6.9874, 3.7617) -> (-6.8857, 3.7109)
  line L534 (-7.0382, 3.7616) -> (-6.9874, 3.7617)
  line L535 (-6.8349, 3.6602) -> (-6.784, 3.5611)
  line L536 (-6.784, 3.5611) -> (-6.7839, 3.3579)
  line L537 (-6.7839, 3.3579) -> (-6.8346, 3.2563)
  line L538 (-6.8346, 3.2563) -> (-6.8853, 3.208)
  line L539 (-6.8853, 3.208) -> (-6.9869, 3.1571)
  line L540 (-6.9869, 3.1571) -> (-7.086, 3.1571)
  line L541 (-7.086, 3.1571) -> (-7.1876, 3.2078)
  line L542 (-7.1876, 3.2078) -> (-7.3401, 3.3067)
  line L543 (-7.3401, 3.3067) -> (-7.8434, 3.8118)
  line L544 (-7.8434, 3.8118) -> (-7.8429, 3.1057)
  line L545 (-7.1365, 2.7633) -> (-7.8426, 2.7628)
  line L546 (-7.3397, 2.7632) -> (-7.1872, 2.6109)
  line L547 (-7.1872, 2.6109) -> (-7.1363, 2.5119)
  line L548 (-7.1363, 2.5119) -> (-7.1362, 2.3595)
  line L549 (-7.1362, 2.3595) -> (-7.1869, 2.2578)
  line L550 (-7.1869, 2.2578) -> (-7.3393, 2.2069)
  line L551 (-7.3393, 2.2069) -> (-7.8422, 2.2065)
  line L552 (-7.3393, 2.2069) -> (-7.1868, 2.0572)
  line L553 (-7.1868, 2.0572) -> (-7.1359, 1.9556)
  line L554 (-7.1359, 1.9556) -> (-7.1358, 1.8057)
  line L555 (-7.1358, 1.8057) -> (-7.1865, 1.7041)
  line L556 (-7.1865, 1.7041) -> (-7.3389, 1.6532)
  line L557 (-7.3389, 1.6532) -> (-7.8418, 1.6528)
  line L558 (-6.7824, 1.3107) -> (-6.8331, 1.2599)
  line L559 (-6.8331, 1.2599) -> (-6.7823, 1.2091)
  line L560 (-6.7823, 1.2091) -> (-6.7341, 1.2599)
  line L561 (-6.7341, 1.2599) -> (-6.7824, 1.3107)
  line L562 (-7.1354, 1.2596) -> (-7.8415, 1.2591)
  line L563 (-6.782, 0.8662) -> (-7.8412, 0.8654)
  line L564 (0.127, -81.0262) -> (-10.7249, -81.0341)
  line L565 (0, 91.9482) -> (-10.8519, 91.9402)
  line L566 (-8.1849, -81.0323) -> (-8.3827, -80.2964)
  line L567 (-8.1849, -81.0323) -> (-7.9883, -80.2961)
  line L568 (-8.3119, 91.9421) -> (-8.5086, 91.2059)
  line L569 (-8.3119, 91.9421) -> (-8.1142, 91.2062)
  line L570 (-8.1849, -81.0323) -> (-8.245, 0.8143)
  line L571 (-8.2518, 10.0955) -> (-8.3119, 91.9421)
  line L572 (26.67, 89.8753) -> (3.556, 89.8753)
  line L573 (3.556, 89.8753) -> (3.5854, 36.5353)
  line L574 (3.5854, 36.5353) -> (26.67, 36.5353)
  line L575 (26.67, 36.5353) -> (26.67, 89.8753)
  line L576 (3.81, 46.6953) -> (3.81, 88.6053)
  line L577 (3.81, 88.6053) -> (5.08, 89.8753)
  line L578 (5.08, 89.8753) -> (26.67, 89.8753)
  line L579 (26.67, 89.8753) -> (26.67, 46.6953)
  line L580 (19.05, 89.8753) -> (19.05, 79.7153)
  line L581 (19.05, 79.7153) -> (11.43, 79.7153)
  line L582 (11.43, 79.7153) -> (11.43, 89.8753)
  line L583 (11.43, 89.8753) -> (19.05, 89.8753)
  line L584 (26.67, 36.5353) -> (3.81, 36.5353)
  line L585 (26.67, 89.8753) -> (3.556, 89.8753)
  line L586 (3.556, 89.8753) -> (3.5854, 36.5353)
  line L587 (3.5854, 36.5353) -> (26.67, 36.5353)
  line L588 (26.67, 36.5353) -> (26.67, 89.8753)
  line L589 (3.81, 46.6953) -> (3.81, 88.6053)
  line L590 (3.81, 88.6053) -> (5.08, 89.8753)
  line L591 (5.08, 89.8753) -> (26.67, 89.8753)
  line L592 (26.67, 89.8753) -> (26.67, 46.6953)
  line L593 (19.05, 89.8753) -> (19.05, 79.7153)
  line L594 (19.05, 79.7153) -> (11.43, 79.7153)
  line L595 (11.43, 79.7153) -> (11.43, 89.8753)
  line L596 (11.43, 89.8753) -> (19.05, 89.8753)
  line L597 (26.67, 36.5353) -> (3.81, 36.5353)
  line L598 (6.0536, 86.9309) -> (5.8719, 87.1809)
  line L599 (6.3475, 86.8354) -> (6.0536, 86.9309)
  line L600 (5.8719, 87.1809) -> (5.8719, 87.4899)
  line L601 (5.8719, 87.4899) -> (6.0536, 87.7399)
  line L602 (6.0536, 87.7399) -> (6.3475, 87.8354)
  line L603 (6.3475, 87.8354) -> (6.3526, 87.8354)
  line L604 (6.3526, 87.8354) -> (6.6464, 87.7399)
  line L605 (6.6464, 87.7399) -> (6.8281, 87.4899)
  line L606 (6.8281, 87.4899) -> (6.8281, 87.1809)
  line L607 (6.8281, 87.1809) -> (6.6464, 86.9309)
  line L608 (6.6464, 86.9309) -> (6.3526, 86.8354)
  line L609 (6.3526, 86.8354) -> (6.3475, 86.8354)
  line L610 (6.3475, 84.2954) -> (6.0536, 84.3909)
  line L611 (6.0536, 84.3909) -> (5.8719, 84.6409)
  line L612 (5.8719, 84.6409) -> (5.8719, 84.9499)
  line L613 (5.8719, 84.9499) -> (6.0536, 85.1999)
  line L614 (6.0536, 85.1999) -> (6.3475, 85.2954)
  line L615 (6.3475, 85.2954) -> (6.3526, 85.2954)
  line L616 (6.3526, 85.2954) -> (6.6464, 85.1999)
  line L617 (6.6464, 85.1999) -> (6.8281, 84.9499)
  line L618 (6.8281, 84.9499) -> (6.8281, 84.6409)
  line L619 (6.8281, 84.6409) -> (6.6464, 84.3909)
  line L620 (6.6464, 84.3909) -> (6.3526, 84.2954)
  line L621 (6.3526, 84.2954) -> (6.3475, 84.2954)
  line L622 (6.3526, 82.7554) -> (6.6464, 82.6599)
  line L623 (6.3475, 81.7554) -> (6.0536, 81.8509)
  line L624 (6.6464, 81.8509) -> (6.3526, 81.7554)
  line L625 (6.8281, 82.1009) -> (6.6464, 81.8509)
  line L626 (6.8281, 82.4099) -> (6.8281, 82.1009)
  line L627 (6.6464, 82.6599) -> (6.8281, 82.4099)
  line L628 (6.3526, 81.7554) -> (6.3475, 81.7554)
  line L629 (6.3475, 82.7554) -> (6.3526, 82.7554)
  line L630 (6.0536, 82.6599) -> (6.3475, 82.7554)
  line L631 (5.8719, 82.4099) -> (6.0536, 82.6599)
  line L632 (5.8719, 82.1009) -> (5.8719, 82.4099)
  line L633 (6.0536, 81.8509) -> (5.8719, 82.1009)
  line L634 (6.3526, 79.2154) -> (6.3475, 79.2154)
  line L635 (6.0536, 79.3109) -> (5.8719, 79.5609)
  line L636 (5.8719, 79.5609) -> (5.8719, 79.8699)
  line L637 (5.8719, 79.8699) -> (6.0536, 80.1199)
  line L638 (6.3475, 79.2154) -> (6.0536, 79.3109)
  line L639 (6.0536, 80.1199) -> (6.3475, 80.2154)
  line L640 (6.3475, 80.2154) -> (6.3526, 80.2154)
  line L641 (6.3526, 80.2154) -> (6.6464, 80.1199)
  line L642 (6.6464, 80.1199) -> (6.8281, 79.8699)
  line L643 (6.8281, 79.8699) -> (6.8281, 79.5609)
  line L644 (6.8281, 79.5609) -> (6.6464, 79.3109)
  line L645 (6.6464, 79.3109) -> (6.3526, 79.2154)
  line L646 (6.3475, 76.6754) -> (6.0536, 76.7709)
  line L647 (6.0536, 76.7709) -> (5.8719, 77.0209)
  line L648 (5.8719, 77.3299) -> (6.0536, 77.5799)
  line L649 (6.0536, 77.5799) -> (6.3475, 77.6754)
  line L650 (6.3475, 77.6754) -> (6.3526, 77.6754)
  line L651 (6.3526, 77.6754) -> (6.6464, 77.5799)
  line L652 (6.6464, 77.5799) -> (6.8281, 77.3299)
  line L653 (6.8281, 77.3299) -> (6.8281, 77.0209)
  line L654 (6.8281, 77.0209) -> (6.6464, 76.7709)
  line L655 (6.6464, 76.7709) -> (6.3526, 76.6754)
  line L656 (6.3526, 76.6754) -> (6.3475, 76.6754)
  line L657 (5.8719, 77.0209) -> (5.8719, 77.3299)
  line L658 (6.0536, 75.0399) -> (6.3475, 75.1354)
  line L659 (5.8719, 74.7899) -> (6.0536, 75.0399)
  line L660 (5.8719, 74.4808) -> (5.8719, 74.7899)
  line L661 (6.0536, 74.2308) -> (5.8719, 74.4808)
  line L662 (6.3475, 74.1354) -> (6.0536, 74.2308)
  line L663 (6.3526, 75.1354) -> (6.6464, 75.0399)
  line L664 (6.6464, 75.0399) -> (6.8281, 74.7899)
  line L665 (6.8281, 74.7899) -> (6.8281, 74.4808)
  line L666 (6.8281, 74.4808) -> (6.6464, 74.2308)
  line L667 (6.6464, 74.2308) -> (6.3526, 74.1354)
  line L668 (6.3526, 74.1354) -> (6.3475, 74.1354)
  line L669 (6.3475, 75.1354) -> (6.3526, 75.1354)
  line L670 (6.3526, 71.5954) -> (6.3475, 71.5954)
  line L671 (6.3475, 71.5954) -> (6.0536, 71.6908)
  line L672 (6.0536, 71.6908) -> (5.8719, 71.9408)
  line L673 (5.8719, 71.9408) -> (5.8719, 72.2499)
  line L674 (5.8719, 72.2499) -> (6.0536, 72.4999)
  line L675 (6.0536, 72.4999) -> (6.3475, 72.5954)
  line L676 (6.3475, 72.5954) -> (6.3526, 72.5954)
  line L677 (6.3526, 72.5954) -> (6.6464, 72.4999)
  line L678 (6.6464, 72.4999) -> (6.8281, 72.2499)
  line L679 (6.8281, 72.2499) -> (6.8281, 71.9408)
  line L680 (6.8281, 71.9408) -> (6.6464, 71.6908)
  line L681 (6.6464, 71.6908) -> (6.3526, 71.5954)
  line L682 (6.6464, 69.9599) -> (6.8281, 69.7099)
  line L683 (6.0536, 69.1508) -> (5.8719, 69.4008)
  line L684 (6.3526, 69.0553) -> (6.3475, 69.0553)
  line L685 (6.6464, 69.1508) -> (6.3526, 69.0553)
  line L686 (6.8281, 69.4008) -> (6.6464, 69.1508)
  line L687 (6.8281, 69.7099) -> (6.8281, 69.4008)
  line L688 (6.3475, 69.0553) -> (6.0536, 69.1508)
  line L689 (6.3526, 70.0553) -> (6.6464, 69.9599)
  line L690 (6.3475, 70.0553) -> (6.3526, 70.0553)
  line L691 (6.0536, 69.9599) -> (6.3475, 70.0553)
  line L692 (5.8719, 69.7099) -> (6.0536, 69.9599)
  line L693 (5.8719, 69.4008) -> (5.8719, 69.7099)
  line L694 (6.3475, 66.5153) -> (6.0536, 66.6108)
  line L695 (6.0536, 66.6108) -> (5.8719, 66.8608)
  line L696 (5.8719, 66.8608) -> (5.8719, 67.1699)
  line L697 (5.8719, 67.1699) -> (6.0536, 67.4199)
  line L698 (6.0536, 67.4199) -> (6.3475, 67.5153)
  line L699 (6.3475, 67.5153) -> (6.3526, 67.5153)
  line L700 (6.3526, 67.5153) -> (6.6464, 67.4199)
  line L701 (6.6464, 67.4199) -> (6.8281, 67.1699)
  line L702 (6.8281, 67.1699) -> (6.8281, 66.8608)
  line L703 (6.8281, 66.8608) -> (6.6464, 66.6108)
  line L704 (6.6464, 66.6108) -> (6.3526, 66.5153)
  line L705 (6.3526, 66.5153) -> (6.3475, 66.5153)
  line L706 (5.8719, 64.3208) -> (5.8719, 64.6298)
  line L707 (6.3475, 63.9753) -> (6.0536, 64.0708)
  line L708 (5.8719, 64.6298) -> (6.0536, 64.8798)
  line L709 (6.0536, 64.8798) -> (6.3475, 64.9753)
  line L710 (6.3475, 64.9753) -> (6.3526, 64.9753)
  line L711 (6.3526, 64.9753) -> (6.6464, 64.8798)
  line L712 (6.6464, 64.8798) -> (6.8281, 64.6298)
  line L713 (6.8281, 64.6298) -> (6.8281, 64.3208)
  line L714 (6.8281, 64.3208) -> (6.6464, 64.0708)
  line L715 (6.6464, 64.0708) -> (6.3526, 63.9753)
  line L716 (6.3526, 63.9753) -> (6.3475, 63.9753)
  line L717 (6.0536, 64.0708) -> (5.8719, 64.3208)
  line L718 (6.0536, 62.3398) -> (6.3475, 62.4353)
  line L719 (6.3526, 62.4353) -> (6.6464, 62.3398)
  line L720 (6.6464, 62.3398) -> (6.8281, 62.0898)
  line L721 (6.8281, 62.0898) -> (6.8281, 61.7808)
  line L722 (6.8281, 61.7808) -> (6.6464, 61.5308)
  line L723 (6.6464, 61.5308) -> (6.3526, 61.4353)
  line L724 (6.3526, 61.4353) -> (6.3475, 61.4353)
  line L725 (5.8719, 62.0898) -> (6.0536, 62.3398)
  line L726 (6.3475, 62.4353) -> (6.3526, 62.4353)
  line L727 (5.8719, 61.7808) -> (5.8719, 62.0898)
  line L728 (6.0536, 61.5308) -> (5.8719, 61.7808)
  line L729 (6.3475, 61.4353) -> (6.0536, 61.5308)
  line L730 (6.3526, 58.8953) -> (6.3475, 58.8953)
  line L731 (6.3475, 58.8953) -> (6.0536, 58.9908)
  line L732 (6.0536, 58.9908) -> (5.8719, 59.2408)
  line L733 (5.8719, 59.2408) -> (5.8719, 59.5498)
  line L734 (5.8719, 59.5498) -> (6.0536, 59.7998)
  line L735 (6.0536, 59.7998) -> (6.3475, 59.8953)
  line L736 (6.3475, 59.8953) -> (6.3526, 59.8953)
  line L737 (6.3526, 59.8953) -> (6.6464, 59.7998)
  line L738 (6.6464, 59.7998) -> (6.8281, 59.5498)
  line L739 (6.8281, 59.5498) -> (6.8281, 59.2408)
  line L740 (6.8281, 59.2408) -> (6.6464, 58.9908)
  line L741 (6.6464, 58.9908) -> (6.3526, 58.8953)
  line L742 (6.8281, 57.0098) -> (6.8281, 56.7008)
  line L743 (5.8719, 56.7008) -> (5.8719, 57.0098)
  line L744 (6.3475, 56.3553) -> (6.0536, 56.4508)
  line L745 (6.3526, 56.3553) -> (6.3475, 56.3553)
  line L746 (6.6464, 56.4508) -> (6.3526, 56.3553)
  line L747 (6.8281, 56.7008) -> (6.6464, 56.4508)
  line L748 (6.0536, 56.4508) -> (5.8719, 56.7008)
  line L749 (6.6464, 57.2598) -> (6.8281, 57.0098)
  line L750 (6.3526, 57.3553) -> (6.6464, 57.2598)
  line L751 (6.3475, 57.3553) -> (6.3526, 57.3553)
  line L752 (6.0536, 57.2598) -> (6.3475, 57.3553)
  line L753 (5.8719, 57.0098) -> (6.0536, 57.2598)
  line L754 (6.3475, 53.8153) -> (6.0536, 53.9108)
  line L755 (6.0536, 53.9108) -> (5.8719, 54.1608)
  line L756 (5.8719, 54.1608) -> (5.8719, 54.4698)
  line L757 (5.8719, 54.4698) -> (6.0536, 54.7198)
  line L758 (6.0536, 54.7198) -> (6.3475, 54.8153)
  line L759 (6.3475, 54.8153) -> (6.3526, 54.8153)
  line L760 (6.3526, 54.8153) -> (6.6464, 54.7198)
  line L761 (6.6464, 54.7198) -> (6.8281, 54.4698)
  line L762 (6.8281, 54.4698) -> (6.8281, 54.1608)
  line L763 (6.8281, 54.1608) -> (6.6464, 53.9108)
  line L764 (6.6464, 53.9108) -> (6.3526, 53.8153)
  line L765 (6.3526, 53.8153) -> (6.3475, 53.8153)
  line L766 (5.8719, 51.9298) -> (6.0536, 52.1798)
  line L767 (5.8719, 51.6208) -> (5.8719, 51.9298)
  line L768 (6.3475, 51.2753) -> (6.0536, 51.3708)
  line L769 (6.0536, 52.1798) -> (6.3475, 52.2753)
  line L770 (6.3475, 52.2753) -> (6.3526, 52.2753)
  line L771 (6.3526, 52.2753) -> (6.6464, 52.1798)
  line L772 (6.6464, 52.1798) -> (6.8281, 51.9298)
  line L773 (6.8281, 51.9298) -> (6.8281, 51.6208)
  line L774 (6.8281, 51.6208) -> (6.6464, 51.3708)
  line L775 (6.6464, 51.3708) -> (6.3526, 51.2753)
  line L776 (6.3526, 51.2753) -> (6.3475, 51.2753)
  line L777 (6.0536, 51.3708) -> (5.8719, 51.6208)
  line L778 (6.0536, 49.6398) -> (6.3475, 49.7353)
  line L779 (6.0536, 48.8308) -> (5.8719, 49.0808)
  line L780 (6.6464, 49.6398) -> (6.8281, 49.3898)
  line L781 (6.8281, 49.3898) -> (6.8281, 49.0808)
  line L782 (5.8719, 49.3898) -> (6.0536, 49.6398)
  line L783 (6.3475, 49.7353) -> (6.3526, 49.7353)
  line L784 (5.8719, 49.0808) -> (5.8719, 49.3898)
  line L785 (6.8281, 49.0808) -> (6.6464, 48.8308)
  line L786 (6.6464, 48.8308) -> (6.3526, 48.7353)
  line L787 (6.3526, 48.7353) -> (6.3475, 48.7353)
  line L788 (6.3526, 49.7353) -> (6.6464, 49.6398)
  line L789 (6.3475, 48.7353) -> (6.0536, 48.8308)
  line L790 (6.3452, 46.1991) -> (6.3401, 46.1991)
  line L791 (6.3401, 46.1991) -> (6.0462, 46.2946)
  line L792 (6.0462, 46.2946) -> (5.8646, 46.5446)
  line L793 (5.8646, 46.5446) -> (5.8646, 46.8536)
  line L794 (5.8646, 46.8536) -> (6.0462, 47.1036)
  line L795 (6.0462, 47.1036) -> (6.3401, 47.1991)
  line L796 (6.3401, 47.1991) -> (6.3452, 47.1991)
  line L797 (6.3452, 47.1991) -> (6.6391, 47.1036)
  line L798 (6.6391, 47.1036) -> (6.8207, 46.8536)
  line L799 (6.8207, 46.8536) -> (6.8207, 46.5446)
  line L800 (6.8207, 46.5446) -> (6.6391, 46.2946)
  line L801 (6.6391, 46.2946) -> (6.3452, 46.1991)
  line L802 (6.6464, 44.5598) -> (6.8281, 44.3098)
  line L803 (5.8719, 44.0008) -> (5.8719, 44.3098)
  line L804 (6.3526, 43.6553) -> (6.3475, 43.6553)
  line L805 (6.6464, 43.7508) -> (6.3526, 43.6553)